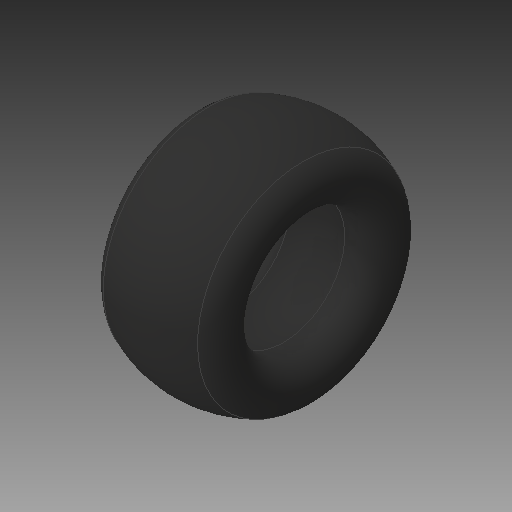
# Autodesk Inventor part: Шина
Saved by Autodesk Inventor 2019 (Build 230136000, 136)
## iProperties
Part Number: Шина
Material: Типовые
Document SubType Name: Modeling
Designer: sbnnl
Density: 1 g/cm^3
Appearance: Резина — черная
Author: sbnnl
Autodesk Inventor part; units mm, degrees
ref_plane "YZ Plane" through (0, 0, 0) normal (1, 0, 0) x (0, 1, 0)
ref_plane "XZ Plane" through (0, 0, 0) normal (0, 1, 0) x (-1, 0, 0)
ref_plane "XY Plane" through (0, 0, 0) normal (0, 0, 1) x (1, 0, 0)
sketch "Эскиз1" plane through (0, 0, 0) normal (1, 0, 0) x (0, 1, 0)
  circle A0 centre (0, 0) radius 75
  dimension "d0" = 150
  constraints: 1 centre point, 1 coincident
  measures "d0" diameter of A0
sketch "Эскиз2" plane through (0, 0, 0) normal (0, 0, 1) x (1, 0, 0)
  arc A0 (31.6327, 70.7504) -> (-31.6327, 70.7504) centre (0, 0) ccw
  arc A1 (-31.6327, 70.7504) -> (-18.3673, 41.0809) centre (-25, 55.9157) ccw
  arc A2 (18.3673, 41.0809) -> (-18.3673, 41.0809) centre (0, 0) ccw
  line L0 (0, 0) -> (0, 86.1934) construction
  arc A3 (18.3673, 41.0809) -> (31.6327, 70.7504) centre (25, 55.9157) ccw
  line L1 (37.5, 0) -> (37.5, 80.388) construction
  line L2 (-37.5, 80.388) -> (-37.5, 0) construction
  dimension "d1" = 90
  dimension "d2" = 155
  dimension "d3" = 25
  dimension "d4" = 75
  constraints: 8 point on circle, 6 end point, 4 centre point, 2 coincident, 2 tangent, 1 parallel, 1 symmetric about line, 1 vertical, 2 other
  measures "d1" diameter of A2
  measures "d2" diameter of A0
  measures "d3" horizontal distance of A1.centre point (0, 0)
  measures "d4" distance of L1.end L2.start
sweep "Сдвиг1" add profiles "Эскиз2" path "Эскиз1"
